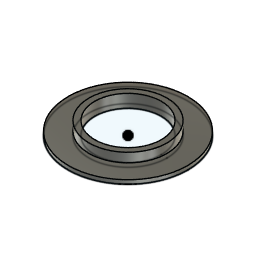
filtre appareil polarisant v1 (Autodesk Fusion 360 design; units mm, degrees)
Autodesk Fusion 360 part; units mm, degrees
sketch "Esquisse1" plane through (0, 0, 0) normal (0, 0, 1) x (1, 0, 0)
  circle A0 centre (0, 0) radius 25.625
  circle A1 centre (0, 0) radius 30
  circle A2 centre (0, 0) radius 46
  dimension "d1" = 51.25
  dimension "d2" = 60
  dimension "d3" = 92
  constraint coincident A0.centre A1.centre
  constraint concentric A0 A1
  measures "d1" diameter of A0
  measures "d2" diameter of A1
  measures "d3" diameter of A2
extrude "Extrusion1" add sketch "Esquisse1" along normal blind 3 contours A2
extrude "Extrusion2" add sketch "Esquisse1" along normal blind 10 contours A1
